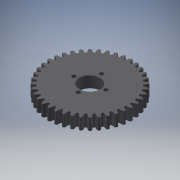
# Autodesk Inventor part: GEAHBB1.0-40-6-A-10_b
Saved by Autodesk Inventor 2016 (Build 200138000, 138)
## iProperties
Category: PARTsolutions
Company: MISUMI
Created: 2016-11-15
Part Number: GEAHBB1.0-40-6-A-10_b
Catalog Web Link: www.cadenas.de
Description: GEAHB1.0, GEAHBB1.0, GEAHBG1.0, GEAHS1.0, GEAB1.0, GEABB1.0, GEABG1.0, GEAS1.0, GEAKB1.0, GEAKBB1.0, GEAKBG1.0, GEAKS1.0_body-Spur Gears - Pressure Angle 20 Degree Module 1.0
Vendor: MISUMI
Document SubType Name: Modeling
Designer: psAdmin
Manufacturer: MISUMI
Mass: 6.98674 g
Surface Area: 39.7208 cm^2
Volume: 6.98674 cm^3
Density: 1 g/cm^3
Material: 一般
Appearance: PSOLRGB-192-192-192
PSOL_IDENT_0: {$CADENAS_DATA\23d-libs\misumi\metric\54_spur_gears\geab10\geab10.prj},466 {VTYP=3D},{NB=GEAHBB1.0-4
PSOL_IDENT_1: 0-6-A-10_b},{LINA=GEAHBB1.0-40-6-A-10},{NN=GEAHB1.0, GEAHBB1.0, GEAHBG1.0, GEAHS1.0, GEAB1.0, GEABB1
PSOL_IDENT_2: .0, GEABG1.0, GEAS1.0, GEAKB1.0, GEAKBB1.0, GEAKBG1.0, GEAKS1.0_body},{DATE=13.09.2016 11:19:06},{GE
PSOL_IDENT_3: OMDATE=13.09.2016 06:08:24},{VERSION=},{LINEID=20},{LINESUBID=-1},{WBVAR=SHS,MAT,ST,NT,B,TS,PS,ALT1,
PSOL_IDENT_4: ALT2,TPC,ALT11,ALT10,BS,ALT4,Z,J,ALT5,Q,R,S,T,ALT9,SRG,ALT6,LFC,LTC,MALT6,ALT7,KFC,KTC,K,ALT3,DIRALT
PSOL_IDENT_5: 3,QFC,QTC,MALT3,ALT8,DIRALT8,ZFC,ZTC,U}  {NB=GEAHBB1.0-40-6-A-10_b},{LINA=GEAHBB1.0-40-6-A-10},{KT=D
PSOL_IDENT_6: UMMY},{PN=GEAHBB1.0-40-6-A-10},{SHS=RH},{TYPE=GEAHBB},{MAT=S45C},{MATALG= 'S45C','S45C Equivalent','
PSOL_IDENT_7: SUS304','SUS304' },{ST=BO},{STALG= '','-','BO','Black Oxide','ENP','Electroless Nickel Plating'},{AC=
PSOL_IDENT_8: -},{MOD=1.0},{NT=40},{NTALG=12,13,14,15,16,17,18,19,20,21,22,23,24,25,26,27,28,29,30,32,34,35,36,38,
PSOL_IDENT_9: 40,42,44,45,46,48,50,52,54,55,56,58,60,62,64,65,66,68,70,72,75,80,84,85,90,95,96,100,110,120},{B=6},
PSOL_IDENT_10: {BALG=6,10},{TS=A},{TSALG='A','A','B','B'},{TSPN=-A},{PS=10},{PSALG='8','8','9','9','10','10','11','
PSOL_IDENT_11: 11','12','12','13','13','14','14','15','15','16','16','17','17'},{P=10.00},{DD=40},{D=42},{G=37.5},{
PSOL_IDENT_12: H=0},{L=0},{LL1=0},{LL2=0},{M=-},{ML=0.000},{ALT1=},{ALT1ALG= '','N/A' },{ALT1PN=},{KC=0},{ALT2=},{A
PSOL_IDENT_13: LT2ALG= '','N/A' },{TPC=N/A},{TPCALG= 'N/A' },{ALT2PN=},{ALT11=},{ALT11ALG= '','N/A' },{ALT11PN=},{D
PSOL_IDENT_14: EG=0},{ALT10=},{ALT10ALG= '','Not applicable' },{BS=0.0},{BSALG=0},{BSMIN=3},{BSMAX=0},{ALT10PN=},{L
PSOL_IDENT_15: L13D=0},{LL23D=0},{LBS=6},{ALT4=},{ALT4ALG='','w/o Stepped Hole','DHL','with DHL (Stepped Hole)','DH
PSOL_IDENT_16: R','with DHR (Stepped Hole)'},{ALT41=1},{ALT42=1},{ALT4PN=},{Z=0},{ZALG=0},{ZPN=},{ZMINL=12},{ZMAXL=
PSOL_IDENT_17: 33},{ZMINR=12},{ZMAXR=33},{J=0.0},{JALG=0},{JPN=},{JMIN=2.0},{JMAX=0.0},{ALT5=},{ALT5ALG= '','Not ap
PSOL_IDENT_18: plicable' },{ALT5PN=},{Q=0},{QALG=0},{QPN=},{QMIN=12},{QMAX=33},{R=0},{RALG=0},{RPN=},{RMIN=12},{RMA
PSOL_IDENT_19: X=33.0},{S=0},{SALG=0},{SPN=},{SMIN=3},{SMAX=0},{T=0},{TALG=0},{TPN=},{TMIN=3},{TMAX=0},{ALT9=},{ALT
PSOL_IDENT_20: 9ALG= '','Not applicable' },{SRG=0.0},{SRGALG=0},{SRGMIN=3.500},{SRGMINALG=3.500},{SRGMAX=0.000},{SR
PSOL_IDENT_21: GMAXALG=0.000},{DD2=0.0},{MM=0.00},{NN=0.00},{DD2ALG=0.000},{MMALG=0.000},{NNALG=0.000},{ALT9PN=},{A
PSOL_IDENT_22: LT6=},{ALT6ALG='','w/o Side Slotted Hole','LFC','with LFC (Side Slotted Hole)','LTC','with LTC (Side
PSOL_IDENT_23: Slotted Hole)'},{ALT6PN=},{LFC=0},{LFCALG=0},{LTC=0},{LTCALG=0},{LPCDMIN=18},{LPCDMAX=30},{MALT6=N/
PSOL_IDENT_24: A},{MALT6ALG= 'N/A' },{C=0.0},{ALT7=},{ALT7ALG= '','w/o Side Through Hole','KFC','with KFC (Side Thr
PSOL_IDENT_25: ough Hole)','KTC','with KTC (Side Through Hole)' },{ALT7PN=},{KFC=0},{KFCALG=[0]},{KTC=0},{KTCALG=[0
PSOL_IDENT_26: ]},{KPCDMIN1=17},{KPCDMAX1=-7},{KPCDMIN2=7},{KPCDMAX2=30},{KPCD=0},{K=0.0},{KALG=[0]},{KALT7L=6},{SC
PSOL_IDENT_27: REW=0},{SCREWL=0},{ALT3=},{ALT3ALG= '','w/o Side Tapped Hole','QFC','with QFC (Side Tapped Hole)','Q
PSOL_IDENT_28: TC','with QTC (Side Tapped Hole)' },{DIRALT3=},{DIRALT3ALG= '','N/A' },{ALT3PN=},{QFC=0},{QFCALG=[0]
PSOL_IDENT_29: },{QTC=0},{QTCALG=[0]},{QPCDMIN1=17},{QPCDMAX1=-7},{QPCDMIN2=7},{QPCDMAX2=30},{CIFMALT3=3},{QPCD=0},
PSOL_IDENT_30: {MALT3=N/A},{MALT3ALG= 'N/A' },{MALT3L=0},{MS1=3},{PITCH=0},{BB=0},{TT=0},{ALT8=},{ALT8ALG= '','Not
PSOL_IDENT_31: applicable' },{DIRALT8=},{DIRALT8ALG= '','N/A' },{ALT8PN=},{ZFC=0},{ZFCALG=[0]},{ZFCMIN=20},{ZFCMAX=
PSOL_IDENT_32: 27},{ZTC=0},{ZTCALG=[0]},{ZPCDMIN1=20},{ZPCDMIN2=11},{ZPCDMAX1=-10},{ZPCDMAX2=27},{ZPCD=0},{U=0},{UA
PSOL_IDENT_33: LG=[0]},{UMAX=0},{UMAX1=0},{UMAX2=0},{UMIN=3},{U1=0.0},{U2=0.0},{F=0.0},{PLANE=5},{BL1=6},{BL2=5.5},
PSOL_IDENT_34: {PCD=0},{SHN=0},{SHDEG1=0},{SHDEG2=0},{PZQRDD2=10},{ALT3LBS=5.5},{D1=2.25},{D2=4.5},{D3=20},{D4=0.1}
PSOL_IDENT_35: ,{D5=6.666667},{D6=6.153846},{D7=0.85},{D8=0.5},{D9=0.824443},{S1=15},{S2=0.5},{KR=18.16}
NN: 0.00
NT: 40
NB: GEAHBB1.0-40-6-A-10_b
NBSYN: $PN._b
LINA: GEAHBB1.0-40-6-A-10
PN: GEAHBB1.0-40-6-A-10
SHS: Round Hole
MAT: S45C Equivalent
ST: Black Oxide
AC: -
MOD: 1.0
B: 6
TS: A
PS: 10
DD: 40
D: 42
G: 37.5
H: 0
L: 0
LL1: 0
LL2: 0
M: -
ALT1: N/A
ALT2: N/A
TPC: N/A
ALT11: N/A
ALT10: Not applicable
BS: 0.0
ALT4: w/o Stepped Hole
Z: 0
J: 0.0
ALT5: Not applicable
Q: 0
R: 0
S: 0
T: 0
ALT9: Not applicable
SRG: 0.0
DD2: 0.0
MM: 0.00
ALT6: w/o Side Slotted Hole
LFC: 0
LTC: 0
MALT6: N/A
C: 0.0
ALT7: w/o Side Through Hole
KFC: 0
KTC: 0
K: 0.0
ALT3: w/o Side Tapped Hole
DIRALT3: N/A
QFC: 0
QTC: 0
MALT3: N/A
ALT8: Not applicable
DIRALT8: N/A
ZFC: 0
ZTC: 0
U: 0
U1: 0.0
U2: 0.0
F: 0.0
SUPPLIER: MISUMI
ARTICLENO: GEAHBB1.0-40-6-A-10_b
BOMINFO: GEAHBB1.0-40-6-A-10
CREATOR: CADENAS GmbH
Title: GEAHBB1.0-40-6-A-10
Author: Cadenas PARTsolutions
Comments: Spur Gears - Pressure Angle 20 Degree Module 1.0
Autodesk Inventor part; units mm, degrees
ref_plane "YZ Plane" through (0, 0, 0) normal (1, 0, 0) x (0, 1, 0)
ref_plane "XZ Plane" through (0, 0, 0) normal (0, 1, 0) x (-1, 0, 0)
ref_plane "XY Plane" through (0, 0, 0) normal (0, 0, 1) x (1, 0, 0)
sketch "Sketch_12" plane through (0, 0, 0) normal (1, 0, 0) x (0, 1, 0)
  line L0 (0, 0) -> (0, 6)
  line L1 (0, 6) -> (20.5, 6)
  line L2 (20.5, 6) -> (26, 4.5263)
  line L3 (26, 4.5263) -> (26, 1.4737)
  line L4 (26, 1.4737) -> (20.5, 0)
  line L5 (20.5, 0) -> (0, 0)
  line L6 (0, 0) -> (0, 6)
  constraints: 14 end point
revolve "Revolution1" add sketch "Sketch_12" angle 360 about axis through (0, 0, 0) along (0, 0, -1)
sketch "Sketch_3" plane through (0, 0, 0) normal (0, 0, 1) x (1, 0, 0)
  circle A0 centre (0, 0) radius 84
  arc A1 (-20.9978, 0.3063) -> (-20.9978, -0.3063) centre (0, 0) ccw
  arc A2 (-20.9978, -0.3063) -> (-20.9426, -0.3942) centre (-20.8978, -0.3048) ccw
  arc A3 (-20.9426, -0.3942) -> (-19.9846, -0.7852) centre (-17.9522, 5.5641) ccw
  arc A4 (-19.9846, -0.7852) -> (-19.8244, -0.8194) centre (-19.7332, 0) ccw
  arc A5 (-19.0802, -0.9496) -> (-19.8244, -0.8194) centre (-20.5105, -6.9349) ccw
  arc A6 (-18.6978, -1.3986) -> (-19.0802, -0.9496) centre (-19.1964, -1.4359) ccw
  arc A7 (-18.6978, -1.3986) -> (-18.6864, -1.5436) centre (0, 0) ccw
  arc A8 (-18.9938, -2.0469) -> (-18.6864, -1.5436) centre (-19.1847, -1.5848) ccw
  arc A9 (-19.7085, -2.2919) -> (-18.9938, -2.0469) centre (-21.3429, 3.6409) ccw
  arc A10 (-19.7085, -2.2919) -> (-19.8614, -2.3507) centre (-19.4903, -3.087) ccw
  arc A11 (-19.8614, -2.3507) -> (-20.7465, -2.8868) centre (-16.8607, -8.3039) ccw
  arc A12 (-20.7465, -2.8868) -> (-20.7872, -2.9823) centre (-20.6882, -2.9681) ccw
  arc A13 (-20.7872, -2.9823) -> (-20.6913, -3.5873) centre (0, 0) ccw
  arc A14 (-20.6913, -3.5873) -> (-20.6231, -3.6655) centre (-20.5928, -3.5702) ccw
  arc A15 (-20.6231, -3.6655) -> (-19.6157, -3.9018) centre (-18.6015, 2.6873) ccw
  arc A16 (-19.6157, -3.9018) -> (-19.4522, -3.9105) centre (-19.4903, -3.087) ccw
  arc A17 (-18.6967, -3.9227) -> (-19.4522, -3.9105) centre (-19.1732, -10.058) ccw
  arc A18 (-18.2488, -4.3063) -> (-18.6967, -3.9227) centre (-18.7354, -4.4212) ccw
  arc A19 (-18.2488, -4.3063) -> (-18.2148, -4.4478) centre (0, 0) ccw
  arc A20 (-18.4397, -4.993) -> (-18.2148, -4.4478) centre (-18.7005, -4.5664) ccw
  arc A21 (-19.1074, -5.3468) -> (-18.4397, -4.993) centre (-21.6497, 0.2573) ccw
  arc A22 (-19.1074, -5.3468) -> (-19.2491, -5.4288) centre (-18.7674, -6.0979) ccw
  arc A23 (-19.2491, -5.4288) -> (-20.0394, -6.0967) centre (-15.3541, -10.8393) ccw
  arc A24 (-20.0394, -6.0967) -> (-20.0647, -6.1974) centre (-19.9692, -6.1679) ccw
  arc A25 (-20.0647, -6.1974) -> (-19.8754, -6.78) centre (0, 0) ccw
  arc A26 (-19.8754, -6.78) -> (-19.7958, -6.8465) centre (-19.7808, -6.7477) ccw
  arc A27 (-19.7958, -6.8465) -> (-18.7638, -6.9223) centre (-18.7929, -0.2557) ccw
  arc A28 (-18.7638, -6.9223) -> (-18.601, -6.9054) centre (-18.7674, -6.0979) ccw
  arc A29 (-17.8529, -6.7992) -> (-18.601, -6.9054) centre (-17.3637, -12.9336) ccw
  arc A30 (-17.3505, -7.108) -> (-17.8529, -6.7992) centre (-17.8131, -7.2976) ccw
  arc A31 (-17.3505, -7.108) -> (-17.2948, -7.2425) centre (0, 0) ccw
  arc A32 (-17.4316, -7.8161) -> (-17.2948, -7.2425) centre (-17.756, -7.4356) ccw
  arc A33 (-18.0357, -8.27) -> (-17.4316, -7.8161) centre (-21.4234, -3.1326) ccw
  arc A34 (-18.0357, -8.27) -> (-18.1629, -8.3732) centre (-17.5824, -8.9587) ccw
  arc A35 (-18.1629, -8.3732) -> (-18.839, -9.1565) centre (-13.4694, -13.1078) ccw
  arc A36 (-18.839, -9.1565) -> (-18.8482, -9.2599) centre (-18.7584, -9.2158) ccw
  arc A37 (-18.8482, -9.2599) -> (-18.5701, -9.8057) centre (0, 0) ccw
  arc A38 (-18.5701, -9.8057) -> (-18.4811, -9.859) centre (-18.4817, -9.759) ccw
  arc A39 (-18.4811, -9.859) -> (-17.4499, -9.7724) centre (-18.5215, -3.1924) ccw
  arc A40 (-17.4499, -9.7724) -> (-17.2917, -9.7302) centre (-17.5824, -8.9587) ccw
  arc A41 (-16.5695, -9.5083) -> (-17.2917, -9.7302) centre (-15.1267, -15.4906) ccw
  arc A42 (-16.0249, -9.7347) -> (-16.5695, -9.5083) centre (-16.4522, -9.9943) ccw
  arc A43 (-16.0249, -9.7347) -> (-15.9489, -9.8588) centre (0, 0) ccw
  arc A44 (-15.9943, -10.4468) -> (-15.9489, -9.8588) centre (-16.3742, -10.1217) ccw
  arc A45 (-16.5199, -10.9896) -> (-15.9943, -10.4468) centre (-20.6696, -6.4454) ccw
  arc A46 (-16.5199, -10.9896) -> (-16.6294, -11.1114) centre (-15.9645, -11.5989) ccw
  arc A47 (-16.6294, -11.1114) -> (-17.1747, -11.9909) centre (-11.2531, -15.0535) ccw
  arc A48 (-17.1747, -11.9909) -> (-17.1676, -12.0944) centre (-17.0858, -12.0368) ccw
  arc A49 (-17.1676, -12.0944) -> (-16.8075, -12.59) centre (0, 0) ccw
  arc A50 (-16.8075, -12.59) -> (-16.7112, -12.6287) centre (-16.7275, -12.53) ccw
  arc A51 (-16.7112, -12.6287) -> (-15.7063, -12.3819) centre (-17.7941, -6.0506) ccw
  arc A52 (-15.7063, -12.3819) -> (-15.5567, -12.3154) centre (-15.9645, -11.5989) ccw
  arc A53 (-14.878, -11.9832) -> (-15.5567, -12.3154) centre (-12.5172, -17.6662) ccw
  arc A54 (-14.3048, -12.1217) -> (-14.878, -11.9832) centre (-14.6862, -12.445) ccw
  arc A55 (-14.3048, -12.1217) -> (-14.2103, -12.2324) centre (0, 0) ccw
  arc A56 (-14.1631, -12.8203) -> (-14.2103, -12.2324) centre (-14.5892, -12.5586) ccw
  arc A57 (-14.5974, -13.4386) -> (-14.1631, -12.8203) centre (-19.4068, -9.5995) ccw
  arc A58 (-14.5974, -13.4386) -> (-14.6865, -13.576) centre (-13.9535, -13.9535) ccw
  arc A59 (-14.6865, -13.576) -> (-15.0874, -14.5299) centre (-8.7597, -16.6285) ccw
  arc A60 (-15.0874, -14.5299) -> (-15.0642, -14.6311) centre (-14.9925, -14.5614) ccw
  arc A61 (-15.0642, -14.6311) -> (-14.6311, -15.0642) centre (0, 0) ccw
  arc A62 (-14.6311, -15.0642) -> (-14.5299, -15.0874) centre (-14.5614, -14.9925) ccw
  arc A63 (-14.5299, -15.0874) -> (-13.576, -14.6865) centre (-16.6285, -8.7597) ccw
  arc A64 (-13.576, -14.6865) -> (-13.4386, -14.5974) centre (-13.9535, -13.9535) ccw
  arc A65 (-12.8203, -14.1631) -> (-13.4386, -14.5974) centre (-9.5995, -19.4068) ccw
  arc A66 (-12.2324, -14.2103) -> (-12.8203, -14.1631) centre (-12.5586, -14.5892) ccw
  arc A67 (-12.2324, -14.2103) -> (-12.1217, -14.3048) centre (0, 0) ccw
  arc A68 (-11.9832, -14.878) -> (-12.1217, -14.3048) centre (-12.445, -14.6862) ccw
  arc A69 (-12.3154, -15.5567) -> (-11.9832, -14.878) centre (-17.6662, -12.5172) ccw
  arc A70 (-12.3154, -15.5567) -> (-12.3819, -15.7063) centre (-11.5989, -15.9645) ccw
  arc A71 (-12.3819, -15.7063) -> (-12.6287, -16.7112) centre (-6.0506, -17.7941) ccw
  arc A72 (-12.6287, -16.7112) -> (-12.59, -16.8075) centre (-12.53, -16.7275) ccw
  arc A73 (-12.59, -16.8075) -> (-12.0944, -17.1676) centre (0, 0) ccw
  arc A74 (-12.0944, -17.1676) -> (-11.9909, -17.1747) centre (-12.0368, -17.0858) ccw
  arc A75 (-11.9909, -17.1747) -> (-11.1114, -16.6294) centre (-15.0535, -11.2531) ccw
  arc A76 (-11.1114, -16.6294) -> (-10.9896, -16.5199) centre (-11.5989, -15.9645) ccw
  arc A77 (-10.4468, -15.9943) -> (-10.9896, -16.5199) centre (-6.4454, -20.6696) ccw
  arc A78 (-9.8588, -15.9489) -> (-10.4468, -15.9943) centre (-10.1217, -16.3742) ccw
  arc A79 (-9.8588, -15.9489) -> (-9.7347, -16.0249) centre (0, 0) ccw
  arc A80 (-9.5083, -16.5695) -> (-9.7347, -16.0249) centre (-9.9943, -16.4522) ccw
  arc A81 (-9.7302, -17.2917) -> (-9.5083, -16.5695) centre (-15.4906, -15.1267) ccw
  arc A82 (-9.7302, -17.2917) -> (-9.7724, -17.4499) centre (-8.9587, -17.5824) ccw
  arc A83 (-9.7724, -17.4499) -> (-9.859, -18.4811) centre (-3.1924, -18.5215) ccw
  arc A84 (-9.859, -18.4811) -> (-9.8057, -18.5701) centre (-9.759, -18.4817) ccw
  arc A85 (-9.8057, -18.5701) -> (-9.2599, -18.8482) centre (0, 0) ccw
  arc A86 (-9.2599, -18.8482) -> (-9.1565, -18.839) centre (-9.2158, -18.7584) ccw
  arc A87 (-9.1565, -18.839) -> (-8.3732, -18.1629) centre (-13.1078, -13.4694) ccw
  arc A88 (-8.3732, -18.1629) -> (-8.27, -18.0357) centre (-8.9587, -17.5824) ccw
  arc A89 (-7.8161, -17.4316) -> (-8.27, -18.0357) centre (-3.1326, -21.4234) ccw
  arc A90 (-7.2425, -17.2948) -> (-7.8161, -17.4316) centre (-7.4356, -17.756) ccw
  arc A91 (-7.2425, -17.2948) -> (-7.108, -17.3505) centre (0, 0) ccw
  arc A92 (-6.7992, -17.8529) -> (-7.108, -17.3505) centre (-7.2976, -17.8131) ccw
  arc A93 (-6.9054, -18.601) -> (-6.7992, -17.8529) centre (-12.9336, -17.3637) ccw
  arc A94 (-6.9054, -18.601) -> (-6.9223, -18.7638) centre (-6.0979, -18.7674) ccw
  arc A95 (-6.9223, -18.7638) -> (-6.8465, -19.7958) centre (-0.2557, -18.7929) ccw
  arc A96 (-6.8465, -19.7958) -> (-6.78, -19.8754) centre (-6.7477, -19.7808) ccw
  arc A97 (-6.78, -19.8754) -> (-6.1974, -20.0647) centre (0, 0) ccw
  arc A98 (-6.1974, -20.0647) -> (-6.0967, -20.0394) centre (-6.1679, -19.9692) ccw
  arc A99 (-6.0967, -20.0394) -> (-5.4288, -19.2491) centre (-10.8393, -15.3541) ccw
  arc A100 (-5.4288, -19.2491) -> (-5.3468, -19.1074) centre (-6.0979, -18.7674) ccw
  arc A101 (-4.993, -18.4397) -> (-5.3468, -19.1074) centre (0.2573, -21.6497) ccw
  arc A102 (-4.4478, -18.2148) -> (-4.993, -18.4397) centre (-4.5664, -18.7005) ccw
  arc A103 (-4.4478, -18.2148) -> (-4.3063, -18.2488) centre (0, 0) ccw
  arc A104 (-3.9227, -18.6967) -> (-4.3063, -18.2488) centre (-4.4212, -18.7354) ccw
  arc A105 (-3.9105, -19.4522) -> (-3.9227, -18.6967) centre (-10.058, -19.1732) ccw
  arc A106 (-3.9105, -19.4522) -> (-3.9018, -19.6157) centre (-3.087, -19.4903) ccw
  arc A107 (-3.9018, -19.6157) -> (-3.6655, -20.6231) centre (2.6873, -18.6015) ccw
  arc A108 (-3.6655, -20.6231) -> (-3.5873, -20.6913) centre (-3.5702, -20.5928) ccw
  arc A109 (-3.5873, -20.6913) -> (-2.9823, -20.7872) centre (0, 0) ccw
  arc A110 (-2.9823, -20.7872) -> (-2.8868, -20.7465) centre (-2.9681, -20.6882) ccw
  arc A111 (-2.8868, -20.7465) -> (-2.3507, -19.8614) centre (-8.3039, -16.8607) ccw
  arc A112 (-2.3507, -19.8614) -> (-2.2919, -19.7085) centre (-3.087, -19.4903) ccw
  arc A113 (-2.0469, -18.9938) -> (-2.2919, -19.7085) centre (3.6409, -21.3429) ccw
  arc A114 (-1.5436, -18.6864) -> (-2.0469, -18.9938) centre (-1.5848, -19.1847) ccw
  arc A115 (-1.5436, -18.6864) -> (-1.3986, -18.6978) centre (0, 0) ccw
  arc A116 (-0.9496, -19.0802) -> (-1.3986, -18.6978) centre (-1.4359, -19.1964) ccw
  arc A117 (-0.8194, -19.8244) -> (-0.9496, -19.0802) centre (-6.9349, -20.5105) ccw
  arc A118 (-0.8194, -19.8244) -> (-0.7852, -19.9846) centre (0, -19.7332) ccw
  arc A119 (-0.7852, -19.9846) -> (-0.3942, -20.9426) centre (5.5641, -17.9522) ccw
  arc A120 (-0.3942, -20.9426) -> (-0.3063, -20.9978) centre (-0.3048, -20.8978) ccw
  arc A121 (-0.3063, -20.9978) -> (0.3063, -20.9978) centre (0, 0) ccw
  arc A122 (0.3063, -20.9978) -> (0.3942, -20.9426) centre (0.3048, -20.8978) ccw
  arc A123 (0.3942, -20.9426) -> (0.7852, -19.9846) centre (-5.5641, -17.9522) ccw
  arc A124 (0.7852, -19.9846) -> (0.8194, -19.8244) centre (0, -19.7332) ccw
  arc A125 (0.9496, -19.0802) -> (0.8194, -19.8244) centre (6.9349, -20.5105) ccw
  arc A126 (1.3986, -18.6978) -> (0.9496, -19.0802) centre (1.4359, -19.1964) ccw
  arc A127 (1.3986, -18.6978) -> (1.5436, -18.6864) centre (0, 0) ccw
  arc A128 (2.0469, -18.9938) -> (1.5436, -18.6864) centre (1.5848, -19.1847) ccw
  arc A129 (2.2919, -19.7085) -> (2.0469, -18.9938) centre (-3.6409, -21.3429) ccw
  arc A130 (2.2919, -19.7085) -> (2.3507, -19.8614) centre (3.087, -19.4903) ccw
  arc A131 (2.3507, -19.8614) -> (2.8868, -20.7465) centre (8.3039, -16.8607) ccw
  arc A132 (2.8868, -20.7465) -> (2.9823, -20.7872) centre (2.9681, -20.6882) ccw
  arc A133 (2.9823, -20.7872) -> (3.5873, -20.6913) centre (0, 0) ccw
  arc A134 (3.5873, -20.6913) -> (3.6655, -20.6231) centre (3.5702, -20.5928) ccw
  arc A135 (3.6655, -20.6231) -> (3.9018, -19.6157) centre (-2.6873, -18.6015) ccw
  arc A136 (3.9018, -19.6157) -> (3.9105, -19.4522) centre (3.087, -19.4903) ccw
  arc A137 (3.9227, -18.6967) -> (3.9105, -19.4522) centre (10.058, -19.1732) ccw
  arc A138 (4.3063, -18.2488) -> (3.9227, -18.6967) centre (4.4212, -18.7354) ccw
  arc A139 (4.3063, -18.2488) -> (4.4478, -18.2148) centre (0, 0) ccw
  arc A140 (4.993, -18.4397) -> (4.4478, -18.2148) centre (4.5664, -18.7005) ccw
  arc A141 (5.3468, -19.1074) -> (4.993, -18.4397) centre (-0.2573, -21.6497) ccw
  arc A142 (5.3468, -19.1074) -> (5.4288, -19.2491) centre (6.0979, -18.7674) ccw
  arc A143 (5.4288, -19.2491) -> (6.0967, -20.0394) centre (10.8393, -15.3541) ccw
  arc A144 (6.0967, -20.0394) -> (6.1974, -20.0647) centre (6.1679, -19.9692) ccw
  arc A145 (6.1974, -20.0647) -> (6.78, -19.8754) centre (0, 0) ccw
  arc A146 (6.78, -19.8754) -> (6.8465, -19.7958) centre (6.7477, -19.7808) ccw
  arc A147 (6.8465, -19.7958) -> (6.9223, -18.7638) centre (0.2557, -18.7929) ccw
  arc A148 (6.9223, -18.7638) -> (6.9054, -18.601) centre (6.0979, -18.7674) ccw
  arc A149 (6.7992, -17.8529) -> (6.9054, -18.601) centre (12.9336, -17.3637) ccw
  arc A150 (7.108, -17.3505) -> (6.7992, -17.8529) centre (7.2976, -17.8131) ccw
  arc A151 (7.108, -17.3505) -> (7.2425, -17.2948) centre (0, 0) ccw
  arc A152 (7.8161, -17.4316) -> (7.2425, -17.2948) centre (7.4356, -17.756) ccw
  arc A153 (8.27, -18.0357) -> (7.8161, -17.4316) centre (3.1326, -21.4234) ccw
  arc A154 (8.27, -18.0357) -> (8.3732, -18.1629) centre (8.9587, -17.5824) ccw
  arc A155 (8.3732, -18.1629) -> (9.1565, -18.839) centre (13.1078, -13.4694) ccw
  arc A156 (9.1565, -18.839) -> (9.2599, -18.8482) centre (9.2158, -18.7584) ccw
  arc A157 (9.2599, -18.8482) -> (9.8057, -18.5701) centre (0, 0) ccw
  arc A158 (9.8057, -18.5701) -> (9.859, -18.4811) centre (9.759, -18.4817) ccw
  arc A159 (9.859, -18.4811) -> (9.7724, -17.4499) centre (3.1924, -18.5215) ccw
  arc A160 (9.7724, -17.4499) -> (9.7302, -17.2917) centre (8.9587, -17.5824) ccw
  arc A161 (9.5083, -16.5695) -> (9.7302, -17.2917) centre (15.4906, -15.1267) ccw
  arc A162 (9.7347, -16.0249) -> (9.5083, -16.5695) centre (9.9943, -16.4522) ccw
  arc A163 (9.7347, -16.0249) -> (9.8588, -15.9489) centre (0, 0) ccw
  arc A164 (10.4468, -15.9943) -> (9.8588, -15.9489) centre (10.1217, -16.3742) ccw
  arc A165 (10.9896, -16.5199) -> (10.4468, -15.9943) centre (6.4454, -20.6696) ccw
  arc A166 (10.9896, -16.5199) -> (11.1114, -16.6294) centre (11.5989, -15.9645) ccw
  arc A167 (11.1114, -16.6294) -> (11.9909, -17.1747) centre (15.0535, -11.2531) ccw
  arc A168 (11.9909, -17.1747) -> (12.0944, -17.1676) centre (12.0368, -17.0858) ccw
  arc A169 (12.0944, -17.1676) -> (12.59, -16.8075) centre (0, 0) ccw
  arc A170 (12.59, -16.8075) -> (12.6287, -16.7112) centre (12.53, -16.7275) ccw
  arc A171 (12.6287, -16.7112) -> (12.3819, -15.7063) centre (6.0506, -17.7941) ccw
  arc A172 (12.3819, -15.7063) -> (12.3154, -15.5567) centre (11.5989, -15.9645) ccw
  arc A173 (11.9832, -14.878) -> (12.3154, -15.5567) centre (17.6662, -12.5172) ccw
  arc A174 (12.1217, -14.3048) -> (11.9832, -14.878) centre (12.445, -14.6862) ccw
  arc A175 (12.1217, -14.3048) -> (12.2324, -14.2103) centre (0, 0) ccw
  arc A176 (12.8203, -14.1631) -> (12.2324, -14.2103) centre (12.5586, -14.5892) ccw
  arc A177 (13.4386, -14.5974) -> (12.8203, -14.1631) centre (9.5995, -19.4068) ccw
  arc A178 (13.4386, -14.5974) -> (13.576, -14.6865) centre (13.9535, -13.9535) ccw
  arc A179 (13.576, -14.6865) -> (14.5299, -15.0874) centre (16.6285, -8.7597) ccw
  arc A180 (14.5299, -15.0874) -> (14.6311, -15.0642) centre (14.5614, -14.9925) ccw
  arc A181 (14.6311, -15.0642) -> (15.0642, -14.6311) centre (0, 0) ccw
  arc A182 (15.0642, -14.6311) -> (15.0874, -14.5299) centre (14.9925, -14.5614) ccw
  arc A183 (15.0874, -14.5299) -> (14.6865, -13.576) centre (8.7597, -16.6285) ccw
  arc A184 (14.6865, -13.576) -> (14.5974, -13.4386) centre (13.9535, -13.9535) ccw
  arc A185 (14.1631, -12.8203) -> (14.5974, -13.4386) centre (19.4068, -9.5995) ccw
  arc A186 (14.2103, -12.2324) -> (14.1631, -12.8203) centre (14.5892, -12.5586) ccw
  arc A187 (14.2103, -12.2324) -> (14.3048, -12.1217) centre (0, 0) ccw
  arc A188 (14.878, -11.9832) -> (14.3048, -12.1217) centre (14.6862, -12.445) ccw
  arc A189 (15.5567, -12.3154) -> (14.878, -11.9832) centre (12.5172, -17.6662) ccw
  arc A190 (15.5567, -12.3154) -> (15.7063, -12.3819) centre (15.9645, -11.5989) ccw
  arc A191 (15.7063, -12.3819) -> (16.7112, -12.6287) centre (17.7941, -6.0506) ccw
  arc A192 (16.7112, -12.6287) -> (16.8075, -12.59) centre (16.7275, -12.53) ccw
  arc A193 (16.8075, -12.59) -> (17.1676, -12.0944) centre (0, 0) ccw
  arc A194 (17.1676, -12.0944) -> (17.1747, -11.9909) centre (17.0858, -12.0368) ccw
  arc A195 (17.1747, -11.9909) -> (16.6294, -11.1114) centre (11.2531, -15.0535) ccw
  arc A196 (16.6294, -11.1114) -> (16.5199, -10.9896) centre (15.9645, -11.5989) ccw
  arc A197 (15.9943, -10.4468) -> (16.5199, -10.9896) centre (20.6696, -6.4454) ccw
  arc A198 (15.9489, -9.8588) -> (15.9943, -10.4468) centre (16.3742, -10.1217) ccw
  arc A199 (15.9489, -9.8588) -> (16.0249, -9.7347) centre (0, 0) ccw
  arc A200 (16.5695, -9.5083) -> (16.0249, -9.7347) centre (16.4522, -9.9943) ccw
  arc A201 (17.2917, -9.7302) -> (16.5695, -9.5083) centre (15.1267, -15.4906) ccw
  arc A202 (17.2917, -9.7302) -> (17.4499, -9.7724) centre (17.5824, -8.9587) ccw
  arc A203 (17.4499, -9.7724) -> (18.4811, -9.859) centre (18.5215, -3.1924) ccw
  arc A204 (18.4811, -9.859) -> (18.5701, -9.8057) centre (18.4817, -9.759) ccw
  arc A205 (18.5701, -9.8057) -> (18.8482, -9.2599) centre (0, 0) ccw
  arc A206 (18.8482, -9.2599) -> (18.839, -9.1565) centre (18.7584, -9.2158) ccw
  arc A207 (18.839, -9.1565) -> (18.1629, -8.3732) centre (13.4694, -13.1078) ccw
  arc A208 (18.1629, -8.3732) -> (18.0357, -8.27) centre (17.5824, -8.9587) ccw
  arc A209 (17.4316, -7.8161) -> (18.0357, -8.27) centre (21.4234, -3.1326) ccw
  arc A210 (17.2948, -7.2425) -> (17.4316, -7.8161) centre (17.756, -7.4356) ccw
  arc A211 (17.2948, -7.2425) -> (17.3505, -7.108) centre (0, 0) ccw
  arc A212 (17.8529, -6.7992) -> (17.3505, -7.108) centre (17.8131, -7.2976) ccw
  arc A213 (18.601, -6.9054) -> (17.8529, -6.7992) centre (17.3637, -12.9336) ccw
  arc A214 (18.601, -6.9054) -> (18.7638, -6.9223) centre (18.7674, -6.0979) ccw
  arc A215 (18.7638, -6.9223) -> (19.7958, -6.8465) centre (18.7929, -0.2557) ccw
  arc A216 (19.7958, -6.8465) -> (19.8754, -6.78) centre (19.7808, -6.7477) ccw
  arc A217 (19.8754, -6.78) -> (20.0647, -6.1974) centre (0, 0) ccw
  arc A218 (20.0647, -6.1974) -> (20.0394, -6.0967) centre (19.9692, -6.1679) ccw
  arc A219 (20.0394, -6.0967) -> (19.2491, -5.4288) centre (15.3541, -10.8393) ccw
  arc A220 (19.2491, -5.4288) -> (19.1074, -5.3468) centre (18.7674, -6.0979) ccw
  arc A221 (18.4397, -4.993) -> (19.1074, -5.3468) centre (21.6497, 0.2573) ccw
  arc A222 (18.2148, -4.4478) -> (18.4397, -4.993) centre (18.7005, -4.5664) ccw
  arc A223 (18.2148, -4.4478) -> (18.2488, -4.3063) centre (0, 0) ccw
  arc A224 (18.6967, -3.9227) -> (18.2488, -4.3063) centre (18.7354, -4.4212) ccw
  arc A225 (19.4522, -3.9105) -> (18.6967, -3.9227) centre (19.1732, -10.058) ccw
  arc A226 (19.4522, -3.9105) -> (19.6157, -3.9018) centre (19.4903, -3.087) ccw
  arc A227 (19.6157, -3.9018) -> (20.6231, -3.6655) centre (18.6015, 2.6873) ccw
  arc A228 (20.6231, -3.6655) -> (20.6913, -3.5873) centre (20.5928, -3.5702) ccw
  arc A229 (20.6913, -3.5873) -> (20.7872, -2.9823) centre (0, 0) ccw
  arc A230 (20.7872, -2.9823) -> (20.7465, -2.8868) centre (20.6882, -2.9681) ccw
  arc A231 (20.7465, -2.8868) -> (19.8614, -2.3507) centre (16.8607, -8.3039) ccw
  arc A232 (19.8614, -2.3507) -> (19.7085, -2.2919) centre (19.4903, -3.087) ccw
  arc A233 (18.9938, -2.0469) -> (19.7085, -2.2919) centre (21.3429, 3.6409) ccw
  arc A234 (18.6864, -1.5436) -> (18.9938, -2.0469) centre (19.1847, -1.5848) ccw
  arc A235 (18.6864, -1.5436) -> (18.6978, -1.3986) centre (0, 0) ccw
  arc A236 (19.0802, -0.9496) -> (18.6978, -1.3986) centre (19.1964, -1.4359) ccw
  arc A237 (19.8244, -0.8194) -> (19.0802, -0.9496) centre (20.5105, -6.9349) ccw
  arc A238 (19.8244, -0.8194) -> (19.9846, -0.7852) centre (19.7332, 0) ccw
  arc A239 (19.9846, -0.7852) -> (20.9426, -0.3942) centre (17.9522, 5.5641) ccw
  arc A240 (20.9426, -0.3942) -> (20.9978, -0.3063) centre (20.8978, -0.3048) ccw
  arc A241 (20.9978, -0.3063) -> (20.9978, 0.3063) centre (0, 0) ccw
  arc A242 (20.9978, 0.3063) -> (20.9426, 0.3942) centre (20.8978, 0.3048) ccw
  arc A243 (20.9426, 0.3942) -> (19.9846, 0.7852) centre (17.9522, -5.5641) ccw
  arc A244 (19.9846, 0.7852) -> (19.8244, 0.8194) centre (19.7332, 0) ccw
  arc A245 (19.0802, 0.9496) -> (19.8244, 0.8194) centre (20.5105, 6.9349) ccw
  arc A246 (18.6978, 1.3986) -> (19.0802, 0.9496) centre (19.1964, 1.4359) ccw
  arc A247 (18.6978, 1.3986) -> (18.6864, 1.5436) centre (0, 0) ccw
  arc A248 (18.9938, 2.0469) -> (18.6864, 1.5436) centre (19.1847, 1.5848) ccw
  arc A249 (19.7085, 2.2919) -> (18.9938, 2.0469) centre (21.3429, -3.6409) ccw
  arc A250 (19.7085, 2.2919) -> (19.8614, 2.3507) centre (19.4903, 3.087) ccw
  arc A251 (19.8614, 2.3507) -> (20.7465, 2.8868) centre (16.8607, 8.3039) ccw
  arc A252 (20.7465, 2.8868) -> (20.7872, 2.9823) centre (20.6882, 2.9681) ccw
  arc A253 (20.7872, 2.9823) -> (20.6913, 3.5873) centre (0, 0) ccw
  arc A254 (20.6913, 3.5873) -> (20.6231, 3.6655) centre (20.5928, 3.5702) ccw
  arc A255 (20.6231, 3.6655) -> (19.6157, 3.9018) centre (18.6015, -2.6873) ccw
  arc A256 (19.6157, 3.9018) -> (19.4522, 3.9105) centre (19.4903, 3.087) ccw
  arc A257 (18.6967, 3.9227) -> (19.4522, 3.9105) centre (19.1732, 10.058) ccw
  arc A258 (18.2488, 4.3063) -> (18.6967, 3.9227) centre (18.7354, 4.4212) ccw
  arc A259 (18.2488, 4.3063) -> (18.2148, 4.4478) centre (0, 0) ccw
  arc A260 (18.4397, 4.993) -> (18.2148, 4.4478) centre (18.7005, 4.5664) ccw
  arc A261 (19.1074, 5.3468) -> (18.4397, 4.993) centre (21.6497, -0.2573) ccw
  arc A262 (19.1074, 5.3468) -> (19.2491, 5.4288) centre (18.7674, 6.0979) ccw
  arc A263 (19.2491, 5.4288) -> (20.0394, 6.0967) centre (15.3541, 10.8393) ccw
  arc A264 (20.0394, 6.0967) -> (20.0647, 6.1974) centre (19.9692, 6.1679) ccw
  arc A265 (20.0647, 6.1974) -> (19.8754, 6.78) centre (0, 0) ccw
  arc A266 (19.8754, 6.78) -> (19.7958, 6.8465) centre (19.7808, 6.7477) ccw
  arc A267 (19.7958, 6.8465) -> (18.7638, 6.9223) centre (18.7929, 0.2557) ccw
  arc A268 (18.7638, 6.9223) -> (18.601, 6.9054) centre (18.7674, 6.0979) ccw
  arc A269 (17.8529, 6.7992) -> (18.601, 6.9054) centre (17.3637, 12.9336) ccw
  arc A270 (17.3505, 7.108) -> (17.8529, 6.7992) centre (17.8131, 7.2976) ccw
  arc A271 (17.3505, 7.108) -> (17.2948, 7.2425) centre (0, 0) ccw
  arc A272 (17.4316, 7.8161) -> (17.2948, 7.2425) centre (17.756, 7.4356) ccw
  arc A273 (18.0357, 8.27) -> (17.4316, 7.8161) centre (21.4234, 3.1326) ccw
  arc A274 (18.0357, 8.27) -> (18.1629, 8.3732) centre (17.5824, 8.9587) ccw
  arc A275 (18.1629, 8.3732) -> (18.839, 9.1565) centre (13.4694, 13.1078) ccw
  arc A276 (18.839, 9.1565) -> (18.8482, 9.2599) centre (18.7584, 9.2158) ccw
  arc A277 (18.8482, 9.2599) -> (18.5701, 9.8057) centre (0, 0) ccw
  arc A278 (18.5701, 9.8057) -> (18.4811, 9.859) centre (18.4817, 9.759) ccw
  arc A279 (18.4811, 9.859) -> (17.4499, 9.7724) centre (18.5215, 3.1924) ccw
  arc A280 (17.4499, 9.7724) -> (17.2917, 9.7302) centre (17.5824, 8.9587) ccw
  arc A281 (16.5695, 9.5083) -> (17.2917, 9.7302) centre (15.1267, 15.4906) ccw
  arc A282 (16.0249, 9.7347) -> (16.5695, 9.5083) centre (16.4522, 9.9943) ccw
  arc A283 (16.0249, 9.7347) -> (15.9489, 9.8588) centre (0, 0) ccw
  arc A284 (15.9943, 10.4468) -> (15.9489, 9.8588) centre (16.3742, 10.1217) ccw
  arc A285 (16.5199, 10.9896) -> (15.9943, 10.4468) centre (20.6696, 6.4454) ccw
  arc A286 (16.5199, 10.9896) -> (16.6294, 11.1114) centre (15.9645, 11.5989) ccw
  arc A287 (16.6294, 11.1114) -> (17.1747, 11.9909) centre (11.2531, 15.0535) ccw
  arc A288 (17.1747, 11.9909) -> (17.1676, 12.0944) centre (17.0858, 12.0368) ccw
  arc A289 (17.1676, 12.0944) -> (16.8075, 12.59) centre (0, 0) ccw
  arc A290 (16.8075, 12.59) -> (16.7112, 12.6287) centre (16.7275, 12.53) ccw
  arc A291 (16.7112, 12.6287) -> (15.7063, 12.3819) centre (17.7941, 6.0506) ccw
  arc A292 (15.7063, 12.3819) -> (15.5567, 12.3154) centre (15.9645, 11.5989) ccw
  arc A293 (14.878, 11.9832) -> (15.5567, 12.3154) centre (12.5172, 17.6662) ccw
  arc A294 (14.3048, 12.1217) -> (14.878, 11.9832) centre (14.6862, 12.445) ccw
  arc A295 (14.3048, 12.1217) -> (14.2103, 12.2324) centre (0, 0) ccw
  arc A296 (14.1631, 12.8203) -> (14.2103, 12.2324) centre (14.5892, 12.5586) ccw
  arc A297 (14.5974, 13.4386) -> (14.1631, 12.8203) centre (19.4068, 9.5995) ccw
  arc A298 (14.5974, 13.4386) -> (14.6865, 13.576) centre (13.9535, 13.9535) ccw
  arc A299 (14.6865, 13.576) -> (15.0874, 14.5299) centre (8.7597, 16.6285) ccw
  arc A300 (15.0874, 14.5299) -> (15.0642, 14.6311) centre (14.9925, 14.5614) ccw
  arc A301 (15.0642, 14.6311) -> (14.6311, 15.0642) centre (0, 0) ccw
  arc A302 (14.6311, 15.0642) -> (14.5299, 15.0874) centre (14.5614, 14.9925) ccw
  arc A303 (14.5299, 15.0874) -> (13.576, 14.6865) centre (16.6285, 8.7597) ccw
  arc A304 (13.576, 14.6865) -> (13.4386, 14.5974) centre (13.9535, 13.9535) ccw
  arc A305 (12.8203, 14.1631) -> (13.4386, 14.5974) centre (9.5995, 19.4068) ccw
  arc A306 (12.2324, 14.2103) -> (12.8203, 14.1631) centre (12.5586, 14.5892) ccw
  arc A307 (12.2324, 14.2103) -> (12.1217, 14.3048) centre (0, 0) ccw
  arc A308 (11.9832, 14.878) -> (12.1217, 14.3048) centre (12.445, 14.6862) ccw
  arc A309 (12.3154, 15.5567) -> (11.9832, 14.878) centre (17.6662, 12.5172) ccw
  arc A310 (12.3154, 15.5567) -> (12.3819, 15.7063) centre (11.5989, 15.9645) ccw
  arc A311 (12.3819, 15.7063) -> (12.6287, 16.7112) centre (6.0506, 17.7941) ccw
  arc A312 (12.6287, 16.7112) -> (12.59, 16.8075) centre (12.53, 16.7275) ccw
  arc A313 (12.59, 16.8075) -> (12.0944, 17.1676) centre (0, 0) ccw
  arc A314 (12.0944, 17.1676) -> (11.9909, 17.1747) centre (12.0368, 17.0858) ccw
  arc A315 (11.9909, 17.1747) -> (11.1114, 16.6294) centre (15.0535, 11.2531) ccw
  arc A316 (11.1114, 16.6294) -> (10.9896, 16.5199) centre (11.5989, 15.9645) ccw
  arc A317 (10.4468, 15.9943) -> (10.9896, 16.5199) centre (6.4454, 20.6696) ccw
  arc A318 (9.8588, 15.9489) -> (10.4468, 15.9943) centre (10.1217, 16.3742) ccw
  arc A319 (9.8588, 15.9489) -> (9.7347, 16.0249) centre (0, 0) ccw
  arc A320 (9.5083, 16.5695) -> (9.7347, 16.0249) centre (9.9943, 16.4522) ccw
  arc A321 (9.7302, 17.2917) -> (9.5083, 16.5695) centre (15.4906, 15.1267) ccw
  arc A322 (9.7302, 17.2917) -> (9.7724, 17.4499) centre (8.9587, 17.5824) ccw
  arc A323 (9.7724, 17.4499) -> (9.859, 18.4811) centre (3.1924, 18.5215) ccw
  arc A324 (9.859, 18.4811) -> (9.8057, 18.5701) centre (9.759, 18.4817) ccw
  arc A325 (9.8057, 18.5701) -> (9.2599, 18.8482) centre (0, 0) ccw
  arc A326 (9.2599, 18.8482) -> (9.1565, 18.839) centre (9.2158, 18.7584) ccw
  arc A327 (9.1565, 18.839) -> (8.3732, 18.1629) centre (13.1078, 13.4694) ccw
  arc A328 (8.3732, 18.1629) -> (8.27, 18.0357) centre (8.9587, 17.5824) ccw
  arc A329 (7.8161, 17.4316) -> (8.27, 18.0357) centre (3.1326, 21.4234) ccw
  arc A330 (7.2425, 17.2948) -> (7.8161, 17.4316) centre (7.4356, 17.756) ccw
  arc A331 (7.2425, 17.2948) -> (7.108, 17.3505) centre (0, 0) ccw
  arc A332 (6.7992, 17.8529) -> (7.108, 17.3505) centre (7.2976, 17.8131) ccw
  arc A333 (6.9054, 18.601) -> (6.7992, 17.8529) centre (12.9336, 17.3637) ccw
  arc A334 (6.9054, 18.601) -> (6.9223, 18.7638) centre (6.0979, 18.7674) ccw
  arc A335 (6.9223, 18.7638) -> (6.8465, 19.7958) centre (0.2557, 18.7929) ccw
  arc A336 (6.8465, 19.7958) -> (6.78, 19.8754) centre (6.7477, 19.7808) ccw
  arc A337 (6.78, 19.8754) -> (6.1974, 20.0647) centre (0, 0) ccw
  arc A338 (6.1974, 20.0647) -> (6.0967, 20.0394) centre (6.1679, 19.9692) ccw
  arc A339 (6.0967, 20.0394) -> (5.4288, 19.2491) centre (10.8393, 15.3541) ccw
  arc A340 (5.4288, 19.2491) -> (5.3468, 19.1074) centre (6.0979, 18.7674) ccw
  arc A341 (4.993, 18.4397) -> (5.3468, 19.1074) centre (-0.2573, 21.6497) ccw
  arc A342 (4.4478, 18.2148) -> (4.993, 18.4397) centre (4.5664, 18.7005) ccw
  arc A343 (4.4478, 18.2148) -> (4.3063, 18.2488) centre (0, 0) ccw
  arc A344 (3.9227, 18.6967) -> (4.3063, 18.2488) centre (4.4212, 18.7354) ccw
  arc A345 (3.9105, 19.4522) -> (3.9227, 18.6967) centre (10.058, 19.1732) ccw
  arc A346 (3.9105, 19.4522) -> (3.9018, 19.6157) centre (3.087, 19.4903) ccw
  arc A347 (3.9018, 19.6157) -> (3.6655, 20.6231) centre (-2.6873, 18.6015) ccw
  arc A348 (3.6655, 20.6231) -> (3.5873, 20.6913) centre (3.5702, 20.5928) ccw
  arc A349 (3.5873, 20.6913) -> (2.9823, 20.7872) centre (0, 0) ccw
  arc A350 (2.9823, 20.7872) -> (2.8868, 20.7465) centre (2.9681, 20.6882) ccw
  arc A351 (2.8868, 20.7465) -> (2.3507, 19.8614) centre (8.3039, 16.8607) ccw
  arc A352 (2.3507, 19.8614) -> (2.2919, 19.7085) centre (3.087, 19.4903) ccw
  arc A353 (2.0469, 18.9938) -> (2.2919, 19.7085) centre (-3.6409, 21.3429) ccw
  arc A354 (1.5436, 18.6864) -> (2.0469, 18.9938) centre (1.5848, 19.1847) ccw
  arc A355 (1.5436, 18.6864) -> (1.3986, 18.6978) centre (0, 0) ccw
  arc A356 (0.9496, 19.0802) -> (1.3986, 18.6978) centre (1.4359, 19.1964) ccw
  arc A357 (0.8194, 19.8244) -> (0.9496, 19.0802) centre (6.9349, 20.5105) ccw
  arc A358 (0.8194, 19.8244) -> (0.7852, 19.9846) centre (0, 19.7332) ccw
  arc A359 (0.7852, 19.9846) -> (0.3942, 20.9426) centre (-5.5641, 17.9522) ccw
  arc A360 (0.3942, 20.9426) -> (0.3063, 20.9978) centre (0.3048, 20.8978) ccw
  arc A361 (0.3063, 20.9978) -> (-0.3063, 20.9978) centre (0, 0) ccw
  arc A362 (-0.3063, 20.9978) -> (-0.3942, 20.9426) centre (-0.3048, 20.8978) ccw
  arc A363 (-0.3942, 20.9426) -> (-0.7852, 19.9846) centre (5.5641, 17.9522) ccw
  arc A364 (-0.7852, 19.9846) -> (-0.8194, 19.8244) centre (0, 19.7332) ccw
  arc A365 (-0.9496, 19.0802) -> (-0.8194, 19.8244) centre (-6.9349, 20.5105) ccw
  arc A366 (-1.3986, 18.6978) -> (-0.9496, 19.0802) centre (-1.4359, 19.1964) ccw
  arc A367 (-1.3986, 18.6978) -> (-1.5436, 18.6864) centre (0, 0) ccw
  arc A368 (-2.0469, 18.9938) -> (-1.5436, 18.6864) centre (-1.5848, 19.1847) ccw
  arc A369 (-2.2919, 19.7085) -> (-2.0469, 18.9938) centre (3.6409, 21.3429) ccw
  arc A370 (-2.2919, 19.7085) -> (-2.3507, 19.8614) centre (-3.087, 19.4903) ccw
  arc A371 (-2.3507, 19.8614) -> (-2.8868, 20.7465) centre (-8.3039, 16.8607) ccw
  arc A372 (-2.8868, 20.7465) -> (-2.9823, 20.7872) centre (-2.9681, 20.6882) ccw
  arc A373 (-2.9823, 20.7872) -> (-3.5873, 20.6913) centre (0, 0) ccw
  arc A374 (-3.5873, 20.6913) -> (-3.6655, 20.6231) centre (-3.5702, 20.5928) ccw
  arc A375 (-3.6655, 20.6231) -> (-3.9018, 19.6157) centre (2.6873, 18.6015) ccw
  arc A376 (-3.9018, 19.6157) -> (-3.9105, 19.4522) centre (-3.087, 19.4903) ccw
  arc A377 (-3.9227, 18.6967) -> (-3.9105, 19.4522) centre (-10.058, 19.1732) ccw
  arc A378 (-4.3063, 18.2488) -> (-3.9227, 18.6967) centre (-4.4212, 18.7354) ccw
  arc A379 (-4.3063, 18.2488) -> (-4.4478, 18.2148) centre (0, 0) ccw
  arc A380 (-4.993, 18.4397) -> (-4.4478, 18.2148) centre (-4.5664, 18.7005) ccw
  arc A381 (-5.3468, 19.1074) -> (-4.993, 18.4397) centre (0.2573, 21.6497) ccw
  arc A382 (-5.3468, 19.1074) -> (-5.4288, 19.2491) centre (-6.0979, 18.7674) ccw
  arc A383 (-5.4288, 19.2491) -> (-6.0967, 20.0394) centre (-10.8393, 15.3541) ccw
  arc A384 (-6.0967, 20.0394) -> (-6.1974, 20.0647) centre (-6.1679, 19.9692) ccw
  arc A385 (-6.1974, 20.0647) -> (-6.78, 19.8754) centre (0, 0) ccw
  arc A386 (-6.78, 19.8754) -> (-6.8465, 19.7958) centre (-6.7477, 19.7808) ccw
  arc A387 (-6.8465, 19.7958) -> (-6.9223, 18.7638) centre (-0.2557, 18.7929) ccw
  arc A388 (-6.9223, 18.7638) -> (-6.9054, 18.601) centre (-6.0979, 18.7674) ccw
  arc A389 (-6.7992, 17.8529) -> (-6.9054, 18.601) centre (-12.9336, 17.3637) ccw
  arc A390 (-7.108, 17.3505) -> (-6.7992, 17.8529) centre (-7.2976, 17.8131) ccw
  arc A391 (-7.108, 17.3505) -> (-7.2425, 17.2948) centre (0, 0) ccw
  arc A392 (-7.8161, 17.4316) -> (-7.2425, 17.2948) centre (-7.4356, 17.756) ccw
  arc A393 (-8.27, 18.0357) -> (-7.8161, 17.4316) centre (-3.1326, 21.4234) ccw
  arc A394 (-8.27, 18.0357) -> (-8.3732, 18.1629) centre (-8.9587, 17.5824) ccw
  arc A395 (-8.3732, 18.1629) -> (-9.1565, 18.839) centre (-13.1078, 13.4694) ccw
  arc A396 (-9.1565, 18.839) -> (-9.2599, 18.8482) centre (-9.2158, 18.7584) ccw
  arc A397 (-9.2599, 18.8482) -> (-9.8057, 18.5701) centre (0, 0) ccw
  arc A398 (-9.8057, 18.5701) -> (-9.859, 18.4811) centre (-9.759, 18.4817) ccw
  arc A399 (-9.859, 18.4811) -> (-9.7724, 17.4499) centre (-3.1924, 18.5215) ccw
  arc A400 (-9.7724, 17.4499) -> (-9.7302, 17.2917) centre (-8.9587, 17.5824) ccw
  arc A401 (-9.5083, 16.5695) -> (-9.7302, 17.2917) centre (-15.4906, 15.1267) ccw
  arc A402 (-9.7347, 16.0249) -> (-9.5083, 16.5695) centre (-9.9943, 16.4522) ccw
  arc A403 (-9.7347, 16.0249) -> (-9.8588, 15.9489) centre (0, 0) ccw
  arc A404 (-10.4468, 15.9943) -> (-9.8588, 15.9489) centre (-10.1217, 16.3742) ccw
  arc A405 (-10.9896, 16.5199) -> (-10.4468, 15.9943) centre (-6.4454, 20.6696) ccw
  arc A406 (-10.9896, 16.5199) -> (-11.1114, 16.6294) centre (-11.5989, 15.9645) ccw
  arc A407 (-11.1114, 16.6294) -> (-11.9909, 17.1747) centre (-15.0535, 11.2531) ccw
  arc A408 (-11.9909, 17.1747) -> (-12.0944, 17.1676) centre (-12.0368, 17.0858) ccw
  arc A409 (-12.0944, 17.1676) -> (-12.59, 16.8075) centre (0, 0) ccw
  arc A410 (-12.59, 16.8075) -> (-12.6287, 16.7112) centre (-12.53, 16.7275) ccw
  arc A411 (-12.6287, 16.7112) -> (-12.3819, 15.7063) centre (-6.0506, 17.7941) ccw
  arc A412 (-12.3819, 15.7063) -> (-12.3154, 15.5567) centre (-11.5989, 15.9645) ccw
  arc A413 (-11.9832, 14.878) -> (-12.3154, 15.5567) centre (-17.6662, 12.5172) ccw
  arc A414 (-12.1217, 14.3048) -> (-11.9832, 14.878) centre (-12.445, 14.6862) ccw
  arc A415 (-12.1217, 14.3048) -> (-12.2324, 14.2103) centre (0, 0) ccw
  arc A416 (-12.8203, 14.1631) -> (-12.2324, 14.2103) centre (-12.5586, 14.5892) ccw
  arc A417 (-13.4386, 14.5974) -> (-12.8203, 14.1631) centre (-9.5995, 19.4068) ccw
  arc A418 (-13.4386, 14.5974) -> (-13.576, 14.6865) centre (-13.9535, 13.9535) ccw
  arc A419 (-13.576, 14.6865) -> (-14.5299, 15.0874) centre (-16.6285, 8.7597) ccw
  arc A420 (-14.5299, 15.0874) -> (-14.6311, 15.0642) centre (-14.5614, 14.9925) ccw
  arc A421 (-14.6311, 15.0642) -> (-15.0642, 14.6311) centre (0, 0) ccw
  arc A422 (-15.0642, 14.6311) -> (-15.0874, 14.5299) centre (-14.9925, 14.5614) ccw
  arc A423 (-15.0874, 14.5299) -> (-14.6865, 13.576) centre (-8.7597, 16.6285) ccw
  arc A424 (-14.6865, 13.576) -> (-14.5974, 13.4386) centre (-13.9535, 13.9535) ccw
  arc A425 (-14.1631, 12.8203) -> (-14.5974, 13.4386) centre (-19.4068, 9.5995) ccw
  arc A426 (-14.2103, 12.2324) -> (-14.1631, 12.8203) centre (-14.5892, 12.5586) ccw
  arc A427 (-14.2103, 12.2324) -> (-14.3048, 12.1217) centre (0, 0) ccw
  arc A428 (-14.878, 11.9832) -> (-14.3048, 12.1217) centre (-14.6862, 12.445) ccw
  arc A429 (-15.5567, 12.3154) -> (-14.878, 11.9832) centre (-12.5172, 17.6662) ccw
  arc A430 (-15.5567, 12.3154) -> (-15.7063, 12.3819) centre (-15.9645, 11.5989) ccw
  arc A431 (-15.7063, 12.3819) -> (-16.7112, 12.6287) centre (-17.7941, 6.0506) ccw
  arc A432 (-16.7112, 12.6287) -> (-16.8075, 12.59) centre (-16.7275, 12.53) ccw
  arc A433 (-16.8075, 12.59) -> (-17.1676, 12.0944) centre (0, 0) ccw
  arc A434 (-17.1676, 12.0944) -> (-17.1747, 11.9909) centre (-17.0858, 12.0368) ccw
  arc A435 (-17.1747, 11.9909) -> (-16.6294, 11.1114) centre (-11.2531, 15.0535) ccw
  arc A436 (-16.6294, 11.1114) -> (-16.5199, 10.9896) centre (-15.9645, 11.5989) ccw
  arc A437 (-15.9943, 10.4468) -> (-16.5199, 10.9896) centre (-20.6696, 6.4454) ccw
  arc A438 (-15.9489, 9.8588) -> (-15.9943, 10.4468) centre (-16.3742, 10.1217) ccw
  arc A439 (-15.9489, 9.8588) -> (-16.0249, 9.7347) centre (0, 0) ccw
  arc A440 (-16.5695, 9.5083) -> (-16.0249, 9.7347) centre (-16.4522, 9.9943) ccw
  arc A441 (-17.2917, 9.7302) -> (-16.5695, 9.5083) centre (-15.1267, 15.4906) ccw
  arc A442 (-17.2917, 9.7302) -> (-17.4499, 9.7724) centre (-17.5824, 8.9587) ccw
  arc A443 (-17.4499, 9.7724) -> (-18.4811, 9.859) centre (-18.5215, 3.1924) ccw
  arc A444 (-18.4811, 9.859) -> (-18.5701, 9.8057) centre (-18.4817, 9.759) ccw
  arc A445 (-18.5701, 9.8057) -> (-18.8482, 9.2599) centre (0, 0) ccw
  arc A446 (-18.8482, 9.2599) -> (-18.839, 9.1565) centre (-18.7584, 9.2158) ccw
  arc A447 (-18.839, 9.1565) -> (-18.1629, 8.3732) centre (-13.4694, 13.1078) ccw
  arc A448 (-18.1629, 8.3732) -> (-18.0357, 8.27) centre (-17.5824, 8.9587) ccw
  arc A449 (-17.4316, 7.8161) -> (-18.0357, 8.27) centre (-21.4234, 3.1326) ccw
  arc A450 (-17.2948, 7.2425) -> (-17.4316, 7.8161) centre (-17.756, 7.4356) ccw
  arc A451 (-17.2948, 7.2425) -> (-17.3505, 7.108) centre (0, 0) ccw
  arc A452 (-17.8529, 6.7992) -> (-17.3505, 7.108) centre (-17.8131, 7.2976) ccw
  arc A453 (-18.601, 6.9054) -> (-17.8529, 6.7992) centre (-17.3637, 12.9336) ccw
  arc A454 (-18.601, 6.9054) -> (-18.7638, 6.9223) centre (-18.7674, 6.0979) ccw
  arc A455 (-18.7638, 6.9223) -> (-19.7958, 6.8465) centre (-18.7929, 0.2557) ccw
  arc A456 (-19.7958, 6.8465) -> (-19.8754, 6.78) centre (-19.7808, 6.7477) ccw
  arc A457 (-19.8754, 6.78) -> (-20.0647, 6.1974) centre (0, 0) ccw
  arc A458 (-20.0647, 6.1974) -> (-20.0394, 6.0967) centre (-19.9692, 6.1679) ccw
  arc A459 (-20.0394, 6.0967) -> (-19.2491, 5.4288) centre (-15.3541, 10.8393) ccw
  arc A460 (-19.2491, 5.4288) -> (-19.1074, 5.3468) centre (-18.7674, 6.0979) ccw
  arc A461 (-18.4397, 4.993) -> (-19.1074, 5.3468) centre (-21.6497, -0.2573) ccw
  arc A462 (-18.2148, 4.4478) -> (-18.4397, 4.993) centre (-18.7005, 4.5664) ccw
  arc A463 (-18.2148, 4.4478) -> (-18.2488, 4.3063) centre (0, 0) ccw
  arc A464 (-18.6967, 3.9227) -> (-18.2488, 4.3063) centre (-18.7354, 4.4212) ccw
  arc A465 (-19.4522, 3.9105) -> (-18.6967, 3.9227) centre (-19.1732, 10.058) ccw
  arc A466 (-19.4522, 3.9105) -> (-19.6157, 3.9018) centre (-19.4903, 3.087) ccw
  arc A467 (-19.6157, 3.9018) -> (-20.6231, 3.6655) centre (-18.6015, -2.6873) ccw
  arc A468 (-20.6231, 3.6655) -> (-20.6913, 3.5873) centre (-20.5928, 3.5702) ccw
  arc A469 (-20.6913, 3.5873) -> (-20.7872, 2.9823) centre (0, 0) ccw
  arc A470 (-20.7872, 2.9823) -> (-20.7465, 2.8868) centre (-20.6882, 2.9681) ccw
  arc A471 (-20.7465, 2.8868) -> (-19.8614, 2.3507) centre (-16.8607, 8.3039) ccw
  arc A472 (-19.8614, 2.3507) -> (-19.7085, 2.2919) centre (-19.4903, 3.087) ccw
  arc A473 (-18.9938, 2.0469) -> (-19.7085, 2.2919) centre (-21.3429, -3.6409) ccw
  arc A474 (-18.6864, 1.5436) -> (-18.9938, 2.0469) centre (-19.1847, 1.5848) ccw
  arc A475 (-18.6864, 1.5436) -> (-18.6978, 1.3986) centre (0, 0) ccw
  arc A476 (-19.0802, 0.9496) -> (-18.6978, 1.3986) centre (-19.1964, 1.4359) ccw
  arc A477 (-19.8244, 0.8194) -> (-19.0802, 0.9496) centre (-20.5105, 6.9349) ccw
  arc A478 (-19.8244, 0.8194) -> (-19.9846, 0.7852) centre (-19.7332, 0) ccw
  arc A479 (-19.9846, 0.7852) -> (-20.9426, 0.3942) centre (-17.9522, -5.5641) ccw
  arc A480 (-20.9426, 0.3942) -> (-20.9978, 0.3063) centre (-20.8978, 0.3048) ccw
  constraints: 960 point on circle, 481 centre point
extrude "Extrusion1" cut sketch "Sketch_3" along normal blind 6
sketch "Sketch3" plane through (0, 0, 0) normal (0, 0, -1) x (-1, 0, 0)
  point P0 (0, 0)
hole "Hole1" at (0, 0, 0) direction (0, 0, 1) diameter 10 depth 6
sketch "_____7" plane through (0, 0, 0) normal (1, 0, 0) x (0, 0, -1)
  line L0 (500, 0) -> (-500, 0)
  line L1 (-0.3, 5) -> (0, 5)
  line L2 (0, 5) -> (0, 5.3)
  line L3 (0, 5.3) -> (-0.3, 5)
  constraints: 8 end point
revolve "Revolution2" cut sketch "_____7" angle 360 about axis through (0, 0, -500) along (0, 0, -1)
sketch "_____17" plane through (0, 0, 0) normal (1, 0, 0) x (0, 0, -1)
  line L0 (500, 0) -> (-500, 0)
  line L1 (-6, 5) -> (-5.7, 5)
  line L2 (-5.7, 5) -> (-6, 5.3)
  line L3 (-6, 5.3) -> (-6, 5)
  constraints: 8 end point
revolve "Revolution3" cut sketch "_____17" angle 360 about axis through (0, 0, -500) along (0, 0, -1)
ref_plane "b_XY" through (0, 0, 0) normal (0, 0, 1) x (1, 0, 0)
ref_plane "b_YZ" through (0, 0, 0) normal (1, 0, 0) x (0, 1, 0)
ref_plane "b_ZX" through (0, 0, 0) normal (0, 1, 0) x (0, 0, 1)
ref_plane "turn_around_XY" through (0, 0, 0) normal (-1, 0, 0) x (0, 0, -1)
ref_plane "turn_around_YZ" through (0, 0, 0) normal (0, 0, -1) x (0, -1, 0)
ref_plane "turn_around_ZX" through (0, 0, 0) normal (0, -1, 0) x (-1, 0, 0)
sketch "スケッチ6" plane through (0, 0, 6) normal (0, 0, 1) x (0.9876883, 0.1564345, 0)
  circle A0 centre (0, 0) radius 7
  circle A1 centre (0, 7) radius 1
  circle A2 centre (7, 0) radius 1
  circle A3 centre (-7, 0) radius 1
  circle A4 centre (0, -7) radius 1
  dimension "d13" = 14
  dimension "d14" = 2
  dimension "d15" = 2
  dimension "d16" = 2
  dimension "d17" = 2
  constraints: 5 centre point, 4 point on circle, 1 coincident
  measures "d13" diameter of A0
  measures "d14" diameter of A1
  measures "d15" diameter of A2
  measures "d16" diameter of A3
  measures "d17" diameter of A4
extrude "押し出し2" cut sketch "スケッチ6" against normal blind 6 contours A0 A2 | A0 A2 | A1 A0 | A0 A1 | A4 A0 | A0 A4 | A3 A0 | A0 A3
body "Solid1"
